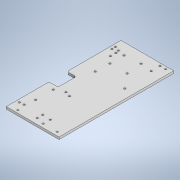
# Autodesk Inventor part: Internal Vert Divider
Saved by Autodesk Inventor 2021 (Build 250183000, 183)
## iProperties
Created: 2020-07-28
Part Number: Internal Vert Divider
Material: Generic
Document SubType Name: Modeling
Designer: jgray
Density: 1 g/cm^3
Appearance: Default
Author: jgray
Autodesk Inventor part; units mm, degrees
ref_plane "YZ Plane" through (0, 0, 0) normal (1, 0, 0) x (0, 1, 0)
ref_plane "XZ Plane" through (0, 0, 0) normal (0, 1, 0) x (-1, 0, 0)
ref_plane "XY Plane" through (0, 0, 0) normal (0, 0, 1) x (1, 0, 0)
sketch "Sketch1" plane through (0, 0, 0) normal (0, 1, 0) x (-1, 0, 0)
  line L0 (0, 0) -> (116.2, 0)
  line L1 (116.2, 0) -> (116.2, -252.75)
  line L2 (116.2, -252.75) -> (0, -252.75)
  line L3 (0, -252.75) -> (0, 0)
  dimension "d0" = 116.2
  dimension "d1" = 252.75
  constraints: 8 end point, 2 parallel, 1 horizontal, 1 perpendicular
  measures "d0" distance of L1.end L2.end
  measures "d1" distance of L0.end L1.end
extrude "Extrusion1" add sketch "Sketch1" along normal blind 5
sketch "Sketch2" plane through (0, 5, 0) normal (0, 1, 0) x (1, 0, 0)
  line L0 (-143.9049, 8) -> (61.1103, 8) construction
  line L1 (-143.9049, 246.75) -> (56.0412, 246.75) construction
  line L2 (-116.2, 0) -> (0, 0) construction
  line L3 (0, 252.75) -> (-116.2, 252.75) construction
  line L4 (0, 0) -> (0, 252.75) construction
  point P0 (-12, 8)
  point P1 (-43, 8)
  point P2 (-12, 246.75)
  point P3 (-24, 246.75)
  dimension "d4" = 8
  dimension "d5" = 6
  dimension "d6" = 12
  dimension "d7" = 12
  dimension "d8" = 12
  dimension "d9" = 31
  constraints: 4 end point, 4 point on line, 2 horizontal
  measures "d4" distance between parallel lines of L2 L0
  measures "d5" distance between parallel lines of L3 L1
  measures "d6" horizontal distance of L2.end point (-12, 8)
  measures "d7" distance from line of L4 point (-12, 246.75)
  measures "d8" distance of point (-24, 246.75) point (-12, 246.75)
  measures "d9" distance of point (-12, 8) point (-43, 8)
hole "Hole1" at (-12, 5, -8) at (-43, 5, -8) at (-12, 5, -246.75) at (-24, 5, -246.75) direction (0, -1, 0) diameter 3.8 end through all
sketch "Sketch3" plane through (0, 5, 0) normal (0, 1, 0) x (1, 0, 0)
  line L0 (-60, 274.5902) -> (-60, -21.6249) construction
  line L1 (0, 0) -> (0, 252.75) construction
  line L2 (0, 252.75) -> (-116.2, 252.75) construction
  line L3 (-116.2, 0) -> (0, 0) projected
  point P0 (-60, 24)
  point P1 (-60, 12)
  dimension "d17" = 60
  dimension "d19" = 12
  dimension "d27" = 12
  constraints: 2 end point, 2 point on line, 1 vertical
  measures "d17" distance between parallel lines of L1 L0
  measures "d19" distance of point (-60, 24) point (-60, 12)
  measures "d27" distance from line of L3 point (-60, 12)
hole "Hole2" at (-60, 5, -24) at (-60, 5, -12) direction (0, -1, 0) diameter 3.8 end through all
sketch "Sketch4" plane through (0, 5, 0) normal (0, 1, 0) x (1, 0, 0)
  line L0 (-150.2588, 199) -> (49.1975, 199) construction
  line L1 (0, 252.75) -> (-116.2, 252.75) construction
  line L2 (-97.7, 275.0226) -> (-97.7, 149.5028) construction
  line L3 (-116.2, 252.75) -> (-116.2, 0) construction
  point P0 (0, 0)
  point P1 (-97.7, 211)
  point P2 (-97.7, 223)
  dimension "d28" = 53.75
  dimension "d29" = 18.5
  dimension "d30" = 12
  dimension "d31" = 24
  constraints: 4 end point, 2 point on line, 1 horizontal, 1 vertical
  measures "d28" distance between parallel lines of L0 L1
  measures "d29" distance between parallel lines of L2 L3
  measures "d30" distance from line of L0 point (-97.7, 211)
  measures "d31" distance from line of L0 point (-97.7, 223)
hole "Hole3" at (-97.7, 5, -211) at (-97.7, 5, -223) direction (0, -1, 0) diameter 3.8 end through all
sketch "Sketch6" plane through (0, 5, 0) normal (0, 1, 0) x (1, 0, 0)
  line L0 (-135.4427, 230.25) -> (59.7258, 230.25) construction
  line L1 (0, 252.75) -> (-116.2, 252.75) construction
  line L2 (-116.2, 252.75) -> (-116.2, 0) construction
  point P0 (0, 0)
  point P1 (-99.5, 230.25)
  point P2 (-49.5, 230.25)
  dimension "d50" = 22.5
  dimension "d51" = 16.7
  dimension "d52" = 66.7
  constraints: 2 end point, 2 point on line, 1 horizontal
  measures "d50" distance between parallel lines of L0 L1
  measures "d51" distance from line of L2 point (-99.5, 230.25)
  measures "d52" distance from line of point (-49.5, 230.25) L2
hole "Hole5" at (-99.5, 5, -230.25) at (-49.5, 5, -230.25) direction (0, -1, 0) diameter 3.8 end through all
sketch "Sketch7" plane through (0, 5, 0) normal (0, 1, 0) x (1, 0, 0)
  line L0 (0, 252.75) -> (-116.2, 252.75) projected
  line L1 (-116.2, 252.75) -> (-116.2, 0) projected
  circle A0 centre (-66.278, 89.237) radius 12
  line L2 (-66.278, 89.237) -> (-96.1481, 98.9825)
  point P0 (0, 0)
  point P1 (-77.6862, 92.9591)
  dimension "d64" = 24
  dimension "d60" = 163.513
  dimension "d61" = 49.922
  dimension "d73" = 71.93
  constraints: 2 end point, 1 coincident, 1 point on line, 3 other
  measures "d60" distance from line of L0 point (-66.278, 89.237)
  measures "d61" distance from line of L1 point (-66.278, 89.237)
  measures "d73" angle of L1 L2
hole "Hole6" at (-66.278, 5, -89.237) at (-77.6862, 5, -92.9591) direction (0, -1, 0) diameter 3.8 end through all
sketch "Sketch8" plane through (0, 5, 0) normal (0, 1, 0) x (1, 0, 0)
  line L0 (-136.1371, 23.25) -> (33.8661, 23.25) construction
  line L1 (-116.2, 0) -> (0, 0) construction
  line L2 (-116.2, 252.75) -> (-116.2, 0) construction
  point P0 (-100.2, 23.25)
  point P1 (-42.7, 23.25)
  dimension "d74" = 23.25
  dimension "d75" = 16
  dimension "d76" = 73.5
  constraints: 2 end point, 2 point on line, 1 horizontal
  measures "d74" distance between parallel lines of L1 L0
  measures "d75" distance from line of L2 point (-100.2, 23.25)
  measures "d76" distance from line of point (-42.7, 23.25) L2
hole "Hole7" at (-100.2, 5, -23.25) at (-42.7, 5, -23.25) direction (0, -1, 0) diameter 3.8 end through all
sketch "Sketch9" plane through (0, 5, 0) normal (0, 1, 0) x (1, 0, 0)
  line L0 (-125.6401, 227.25) -> (33.4538, 227.25) construction
  line L1 (0, 252.75) -> (-116.2, 252.75) projected
  line L2 (0, 0) -> (0, 252.75) projected
  line L3 (-167.8122, 196.25) -> (35.3783, 196.25) construction
  line L4 (-116.2, 252.75) -> (-116.2, 0) projected
  point P0 (-24, 227.25)
  point P1 (-84, 227.25)
  point P2 (-84, 196.25)
  point P3 (-46, 196.25)
  point P4 (-109.5, 226.25)
  dimension "d84" = 25.5
  dimension "d85" = 24
  dimension "d86" = 84
  dimension "d94" = 56.5
  dimension "d95" = 84
  dimension "d96" = 46
  dimension "d97" = 26.5
  dimension "d98" = 6.7
  constraints: 4 end point, 4 point on line, 2 horizontal
  measures "d84" distance between parallel lines of L0 L1
  measures "d85" distance from line of L2 point (-24, 227.25)
  measures "d86" distance from line of L2 point (-84, 227.25)
  measures "d94" distance between parallel lines of L1 L3
  measures "d95" distance from line of point (-84, 196.25) L2
  measures "d96" distance from line of L2 point (-46, 196.25)
  measures "d97" distance from line of L1 point (-109.5, 226.25)
  measures "d98" distance from line of point (-109.5, 226.25) L4
hole "Hole8" at (-24, 5, -227.25) at (-84, 5, -227.25) at (-84, 5, -196.25) at (-46, 5, -196.25) at (-109.5, 5, -226.25) direction (0, -1, 0) diameter 3.8 end through all
sketch "Sketch10" plane through (0, 5, 0) normal (0, 1, 0) x (1, 0, 0)
  line L0 (-109.7, 267.6136) -> (-109.7, -16.6151) construction
  line L1 (-116.2, 252.75) -> (-116.2, 0) construction
  line L2 (0, 252.75) -> (-116.2, 252.75) projected
  point P0 (0, 0)
  point P1 (-109.7, 234)
  point P2 (-109.7, 22.25)
  dimension "d99" = 6.5
  dimension "d100" = 18.75
  dimension "d101" = 211.75
  constraints: 2 end point, 2 point on line, 1 parallel
  measures "d99" distance between parallel lines of L0 L1
  measures "d100" distance from line of L2 point (-109.7, 234)
  measures "d101" distance of point (-109.7, 22.25) point (-109.7, 234)
hole "Hole9" at (-109.7, 5, -234) at (-109.7, 5, -22.25) direction (0, -1, 0) diameter 3.8 end through all
sketch "Sketch11" plane through (0, 5, 0) normal (0, 1, 0) x (1, 0, 0)
  line L0 (-96.7, 85.8638) -> (-96.7, -44.5279) construction
  line L1 (-141.7957, 6) -> (-51.6043, 6) construction
  line L2 (-116.2, 0) -> (0, 0) projected
  line L3 (-116.2, 252.75) -> (-116.2, 0) projected
  point P0 (-96.7, 45)
  point P1 (-96.7, 84)
  point P2 (-96.7, 6)
  dimension "d109" = 6
  dimension "d110" = 19.5
  dimension "d111" = 39
  dimension "d112" = 39
  constraints: 4 end point, 3 point on line, 1 horizontal, 1 midpoint, 1 vertical
  measures "d109" distance between parallel lines of L2 L1
  measures "d110" distance between parallel lines of L0 L3
  measures "d111" distance of point (-96.7, 45) point (-96.7, 6)
  measures "d112" distance of point (-96.7, 84) point (-96.7, 45)
hole "Hole10" at (-96.7, 5, -45) at (-96.7, 5, -84) at (-96.7, 5, -6) direction (0, -1, 0) diameter 3.8 end through all
sketch "Sketch12" plane through (0, 5, 0) normal (0, 1, 0) x (1, 0, 0)
  line L0 (-148.2315, 164.75) -> (24.3981, 164.75) construction
  line L1 (0, 252.75) -> (-116.2, 252.75) projected
  line L2 (0, 0) -> (0, 252.75) projected
  point P0 (-20, 164.75)
  point P1 (-85, 164.75)
  dimension "d120" = 88
  dimension "d121" = 20
  dimension "d122" = 85
  constraints: 2 end point, 2 point on line, 1 horizontal
  measures "d120" distance between parallel lines of L0 L1
  measures "d121" distance from line of L2 point (-20, 164.75)
  measures "d122" distance from line of L2 point (-85, 164.75)
hole "Hole11" at (-20, 5, -164.75) at (-85, 5, -164.75) direction (0, -1, 0) diameter 3.8 end through all
sketch "Sketch13" plane through (0, 5, 0) normal (0, 1, 0) x (1, 0, 0)
  line L0 (-159.8751, 114) -> (39.6093, 114) construction
  line L1 (-116.2, 0) -> (0, 0) construction
  line L2 (-96.2, 94) -> (-136.2, 94)
  line L3 (-136.2, 94) -> (-136.2, 134)
  line L4 (-136.2, 134) -> (-96.2, 134)
  line L5 (-96.2, 134) -> (-96.2, 94)
  line L6 (-116.2, 252.75) -> (-116.2, 0) construction
  line L7 (-96.2, 94) -> (-136.2, 134) construction
  line L8 (-136.2, 94) -> (-96.2, 134) construction
  point P0 (-116.2, 114)
  dimension "d130" = 114
  dimension "d131" = 40
  dimension "d132" = 40
  constraints: 14 end point, 2 horizontal, 2 midpoint, 2 parallel, 2 point on line, 1 perpendicular
  measures "d130" distance between parallel lines of L1 L0
  measures "d131" distance of L3.end L4.end
  measures "d132" distance of L2.end L3.end
extrude "Extrusion2" cut sketch "Sketch13" against normal through all
fillet "Fillet1" radius 4 4 edges at (-116.2, 2.5, -134) (-116.2, 2.5, -94) (-96.2, 2.5, -94) (-96.2, 2.5, -134)
fillet "Fillet2" radius 2 1 edges at (-116.2, 2.5, -252.75)
body "Solid1"
